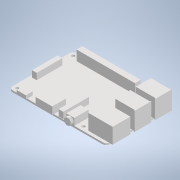
# Autodesk Inventor part: RaspberryPi3B_Mockup
Saved by Autodesk Inventor 2021 (Build 250183000, 183)
## iProperties
Created: 2021-04-19
Part Number: RaspberryPi3B_Mockup
Material: Generic
Document SubType Name: Modeling
Designer: trent
Density: 1 g/cm^3
Appearance: Default
Author: trent
Autodesk Inventor part; units mm, degrees
ref_plane "YZ Plane" through (0, 0, 0) normal (1, 0, 0) x (0, 1, 0)
ref_plane "XZ Plane" through (0, 0, 0) normal (0, 1, 0) x (-1, 0, 0)
ref_plane "XY Plane" through (0, 0, 0) normal (0, 0, 1) x (1, 0, 0)
sketch "Sketch1" plane through (0, 0, 0) normal (0, 1, 0) x (-1, 0, 0)
  line L0 (-3, 0) -> (-82, 0)
  line L1 (-85, -3) -> (-85, -53)
  line L2 (-82, -56) -> (-3, -56)
  line L3 (0, -53) -> (0, -3)
  arc A0 (-3, -56) -> (0, -53) centre (-3, -53) ccw
  arc A1 (0, -3) -> (-3, 0) centre (-3, -3) ccw
  arc A2 (-82, 0) -> (-85, -3) centre (-82, -3) ccw
  arc A3 (-85, -53) -> (-82, -56) centre (-82, -53) ccw
  circle A4 centre (-3.5, -52.5) radius 1.35
  circle A5 centre (-3.5, -3.5) radius 1.35
  circle A6 centre (-61.5, -52.5) radius 1.35
  circle A7 centre (-61.5, -3.5) radius 1.35
  point P0 (0, 0)
  point P1 (-85, -56)
  point P2 (-85, 0)
  point P3 (0, -56)
  dimension "d0" = 85
  dimension "d1" = 56
  dimension "d2" = 3
  dimension "d9" = 2.7
  dimension "d10" = 2.7
  dimension "d15" = 2.7
  dimension "d16" = 2.7
  dimension "d140" = 58
  dimension "d141" = 58
  dimension "d142" = 49
  dimension "d143" = 3.5
  constraints: 8 centre point, 8 end point, 8 point on circle, 8 point on line, 8 tangent, 3 equal radius, 2 parallel, 1 horizontal, 1 perpendicular
  measures "d0" distance of point (-85, -56) point (0, -56)
  measures "d1" distance of point (-85, 0) point (-85, -56)
  measures "d2" radius of A0
  measures "d9" diameter of A4
  measures "d10" diameter of A5
  measures "d15" diameter of A6
  measures "d16" diameter of A7
  measures "d140" distance of A6.centre A4.centre
  measures "d141" distance of A5.centre A7.centre
  measures "d142" distance of A4.centre A5.centre
  measures "d143" distance from line of L0 A5.centre
extrude "Extrusion1" add sketch "Sketch1" along normal blind 1.5
sketch "Sketch2" plane through (0, 1.5, 0) normal (0, 1, 0) x (1, 0, 0)
  circle A0 centre (3.5, 3.5) radius 1.35 projected
  circle A1 centre (3.5, 3.5) radius 3
  circle A2 centre (3.5, 52.5) radius 1.35 projected
  circle A3 centre (3.5, 52.5) radius 3
  circle A4 centre (61.5, 52.5) radius 1.35 projected
  circle A5 centre (61.5, 52.5) radius 3
  circle A6 centre (61.5, 3.5) radius 1.35 projected
  circle A7 centre (61.5, 3.5) radius 3
  point P0 (0, 0)
  dimension "d19" = 6
  dimension "d20" = 6
  dimension "d21" = 6
  dimension "d22" = 6
  constraints: 4 centre point, 4 coincident
  measures "d19" diameter of A1
  measures "d20" diameter of A3
  measures "d21" diameter of A5
  measures "d22" diameter of A7
extrude "Extrusion2" cut sketch "Sketch2" against normal blind 0.001 contours A0 | A1 | A3 | A5 | A6 | A7
sketch "Sketch3" plane through (0, 1.5, 0) normal (0, 1, 0) x (1, 0, 0)
  line L0 (7.25, 55) -> (58.25, 55)
  line L1 (58.25, 55) -> (58.25, 50)
  line L2 (58.25, 50) -> (7.25, 50)
  line L3 (7.25, 50) -> (7.25, 55)
  line L4 (32.75, 55) -> (32.75, 50)
  line L5 (32.75, 52.5) -> (7.25, 52.5)
  line L6 (0, 53) -> (0, 3) projected
  line L7 (82, 56) -> (3, 56) projected
  circle A0 centre (3.5, 52.5) radius 1.35 projected
  point P0 (0, 0)
  dimension "d25" = 51
  dimension "d26" = 5
  dimension "d28" = 25.5
  dimension "d29" = 2.5
  dimension "d30" = 3.5
  dimension "d152" = 7.25
  constraints: 12 end point, 4 midpoint, 2 parallel, 1 horizontal, 1 perpendicular
  measures "d25" distance of L0.start L0.end
  measures "d26" distance of L0.end L1.end
  measures "d28" distance between parallel lines of L4 L3
  measures "d29" distance between parallel lines of L0 L5
  measures "d30" distance between parallel lines of L7 L5
  measures "d152" distance between parallel lines of L6 L3
extrude "Extrusion3" add sketch "Sketch3" along normal blind 8.75 contours L0 L4 L5 L3 | L0 L1 L2 L4 | L5 L4 L2 L3
sketch "Sketch4" plane through (0, 1.5, 0) normal (0, 1, 0) x (1, 0, 0)
  line L0 (1.95, 18.15) -> (6.05, 18.15)
  line L1 (6.05, 18.15) -> (6.05, 40.55)
  line L2 (6.05, 40.55) -> (1.95, 40.55)
  line L3 (1.95, 40.55) -> (1.95, 18.15)
  line L4 (4, 40.55) -> (4, 18.15)
  line L5 (1.95, 29.35) -> (6.05, 29.35)
  line L6 (0, 53) -> (0, 3) projected
  circle A0 centre (3.5, 3.5) radius 1.35 projected
  point P0 (0, 0)
  dimension "d34" = 4.1
  dimension "d35" = 22.4
  dimension "d36" = 4
  dimension "d37" = 24.5
  constraints: 12 end point, 4 midpoint, 2 parallel, 1 horizontal, 1 perpendicular
  measures "d34" distance of L1.end L2.end
  measures "d35" distance of L0.end L1.end
  measures "d36" distance between parallel lines of L6 L4
  measures "d37" distance edge to line of A0 L5
extrude "Extrusion4" add sketch "Sketch4" along normal blind 5.5 contours L3 L5 L4 L0 | L4 L5 L1 L0 | L3 L2 L4 L5 | L4 L2 L1 L5
sketch "Sketch5" plane through (0, 1.5, 0) normal (0, 1, 0) x (1, 0, 0)
  line L0 (7.93, 4.71) -> (15.97, 4.71)
  line L1 (15.97, 4.71) -> (15.97, -1.22)
  line L2 (15.97, -1.22) -> (7.93, -1.22)
  line L3 (7.93, -1.22) -> (7.93, 4.71)
  line L4 (3, 0) -> (82, 0) projected
  line L5 (11.95, -1.22) -> (11.95, 4.71)
  circle A0 centre (3.5, 3.5) radius 1.35 projected
  point P0 (0, 0)
  dimension "d44" = 1.22
  dimension "d45" = 5.93
  dimension "d46" = 8.04
  dimension "d74" = 7.1
  constraints: 10 end point, 2 midpoint, 2 parallel, 1 horizontal, 1 perpendicular
  measures "d44" distance between parallel lines of L2 L4
  measures "d45" distance of L2.end L0.start
  measures "d46" distance of L1.end L2.end
  measures "d74" distance edge to line of A0 L5
extrude "Extrusion5" add sketch "Sketch5" along normal blind 3.2 contours L0 L5 L4 L3 | L0 L1 L4 L5 | L4 L5 L2 L3 | L4 L1 L2 L5
sketch "Sketch6" plane through (0, 1.5, 0) normal (0, 1, 0) x (1, 0, 0)
  line L0 (7.93, -1.22) -> (15.97, -1.22) projected
  line L1 (11.95, -1.22) -> (11.95, 4.71)
  line L2 (7.93, 4.71) -> (15.97, 4.71) projected
  line L3 (24.75, 10.65) -> (39.25, 10.65)
  line L4 (39.25, 10.65) -> (39.25, -1.5)
  line L5 (39.25, -1.5) -> (24.75, -1.5)
  line L6 (24.75, -1.5) -> (24.75, 10.65)
  line L7 (15.97, 0) -> (82, 0) projected
  circle A0 centre (3.5, 3.5) radius 1.35 projected
  line L8 (0, 53) -> (0, 3) projected
  point P0 (0, 0)
  dimension "d144" = 14.5
  dimension "d145" = 12.15
  dimension "d146" = 1.5
  dimension "d153" = 24.75
  constraints: 10 end point, 2 midpoint, 2 parallel, 1 horizontal, 1 perpendicular
  measures "d144" distance of L4.end L5.end
  measures "d145" distance of L3.end L4.end
  measures "d146" distance between parallel lines of L5 L7
  measures "d153" distance between parallel lines of L8 L6
extrude "Extrusion6" add sketch "Sketch6" along normal blind 6.5 contours L3 L4 L7 L6 | L7 L4 L5 L6
sketch "Sketch7" plane through (0, 1.5, 0) normal (0, 1, 0) x (1, 0, 0)
  line L0 (1.95, 40.55) -> (1.95, 18.15) projected
  line L1 (6.05, 18.15) -> (6.05, 40.55) projected
  line L2 (42.95, 22.7) -> (47.05, 22.7)
  line L3 (47.05, 22.7) -> (47.05, 0.3)
  line L4 (47.05, 0.3) -> (42.95, 0.3)
  line L5 (42.95, 0.3) -> (42.95, 22.7)
  line L6 (45, 0.3) -> (45, 22.7)
  line L7 (42.95, 11.5) -> (47.05, 11.5)
  line L8 (0, 53) -> (0, 3) projected
  point P0 (0, 0)
  dimension "d78" = 4.1
  dimension "d80" = 22.4
  dimension "d150" = 45
  constraints: 12 end point, 4 midpoint, 2 parallel, 1 horizontal, 1 perpendicular
  measures "d78" distance of L2.start L2.end
  measures "d80" distance of L0.start L0.end
  measures "d150" distance between parallel lines of L8 L6
extrude "Extrusion7" add sketch "Sketch7" along normal blind 5.5
sketch "Sketch8" plane through (0, 1.5, 0) normal (0, 1, 0) x (1, 0, 0)
  line L0 (50, 0) -> (57, 0)
  line L1 (57, 0) -> (57, 12.5)
  line L2 (57, 12.5) -> (50, 12.5)
  line L3 (50, 12.5) -> (50, 0)
  line L4 (50, 6.25) -> (57, 6.25)
  line L5 (53.5, 0) -> (53.5, 12.5)
  line L6 (3, 0) -> (82, 0) projected
  line L7 (47.05, 0.3) -> (42.95, 0.3) projected
  line L8 (45, 0.3) -> (45, 22.7)
  line L9 (42.95, 22.7) -> (47.05, 22.7) projected
  circle A0 centre (3.5, 3.5) radius 1.35 projected
  line L10 (0, 53) -> (0, 3) projected
  point P0 (0, 0)
  point P1 (43.35, 0)
  dimension "d85" = 7
  dimension "d86" = 12.5
  dimension "d89" = 0
  dimension "d149" = 53.5
  constraints: 14 end point, 6 midpoint, 2 parallel, 1 horizontal, 1 perpendicular
  measures "d85" distance of L1.end L2.end
  measures "d86" distance of L0.end L1.end
  measures "d89" distance between parallel lines of L6 L0
  measures "d149" distance between parallel lines of L10 L5
extrude "Extrusion8" add sketch "Sketch8" along normal blind 6 contours L3 L4 L5 L0 | L5 L4 L1 L0 | L3 L2 L5 L4 | L5 L2 L1 L4
sketch "Sketch9" plane through (3, 0, 0) normal (0, 0, 1) x (1, 0, 0)
  line L0 (54, 7.5) -> (47, 7.5) projected
  line L1 (54, 1.5) -> (54, 7.5) projected
  circle A0 centre (50.5, 4.25) radius 3
  point P0 (-3, 0)
  dimension "d96" = 3.5
  dimension "d97" = 3.25
  dimension "d98" = 6
  constraints: 1 centre point
  measures "d96" distance from line of L1 A0.centre
  measures "d97" distance from line of L0 A0.centre
  measures "d98" diameter of A0
extrude "Extrusion9" add sketch "Sketch9" along normal blind 2.5
sketch "Sketch10" plane through (0, 1.5, 0) normal (0, 1, 0) x (1, 0, 0)
  line L0 (66.65, 18) -> (88, 18)
  line L1 (88, 18) -> (88, 2.5)
  line L2 (88, 2.5) -> (66.65, 2.5)
  line L3 (66.65, 2.5) -> (66.65, 18)
  line L4 (85, 3) -> (85, 53) projected
  line L5 (88, 10.25) -> (66.65, 10.25)
  line L6 (57, 0) -> (82, 0) projected
  point P0 (0, 0)
  dimension "d101" = 21.35
  dimension "d102" = 15.5
  dimension "d103" = 3
  dimension "d104" = 10.25
  constraints: 10 end point, 2 midpoint, 2 parallel, 1 horizontal, 1 perpendicular
  measures "d101" distance of L0.start L0.end
  measures "d102" distance of L2.end L0.start
  measures "d103" distance between parallel lines of L1 L4
  measures "d104" distance between parallel lines of L6 L5
extrude "Extrusion10" add sketch "Sketch10" along normal blind 13.5
sketch "Sketch11" plane through (0, 1.5, 0) normal (0, 1, 0) x (1, 0, 0)
  line L0 (70.3341, 22.43) -> (87.5, 22.43)
  line L1 (88, 2.4833) -> (88, 15.6315)
  line L2 (87.5, 35.57) -> (70.3341, 35.57)
  line L3 (70.3341, 35.57) -> (70.3341, 22.43)
  line L4 (85, 3) -> (85, 53) projected
  line L5 (88, 36.35) -> (87.5, 36.35)
  line L6 (87.5, 21.65) -> (88, 21.65)
  line L7 (88, 21.65) -> (88, 36.35)
  line L8 (87.5, 36.35) -> (87.5, 35.57)
  line L9 (87.5, 22.43) -> (87.5, 21.65)
  line L10 (88, 29) -> (70.3341, 29)
  line L11 (70.3, 40.43) -> (87.5, 40.43)
  line L12 (88, 22.6143) -> (88, 34.7304)
  line L13 (87.5, 53.57) -> (70.3, 53.57)
  line L14 (70.3, 53.57) -> (70.3, 40.43)
  line L15 (88, 54.35) -> (87.5, 54.35)
  line L16 (87.5, 39.65) -> (88, 39.65)
  line L17 (88, 39.65) -> (88, 54.35)
  line L18 (87.5, 54.35) -> (87.5, 53.57)
  line L19 (87.5, 40.43) -> (87.5, 39.65)
  line L20 (88, 47) -> (70.3, 47)
  line L21 (66.65, 2.5) -> (66.65, 18) projected
  line L22 (66.65, 10.25) -> (88, 10.25)
  line L23 (57, 0) -> (82, 0) projected
  point P0 (0, 0)
  point P1 (85, 38)
  point P2 (88, 34.35)
  dimension "d107" = 3
  dimension "d109" = 13.14
  dimension "d113" = 14.7
  dimension "d115" = 13.14
  dimension "d119" = 14.7
  dimension "d123" = 29
  dimension "d125" = 14.7
  dimension "d126" = 3
  dimension "d127" = 3
  dimension "d129" = 2.5
  dimension "d130" = 2.5
  dimension "d131" = 2.5
  dimension "d132" = 14.6659
  dimension "d133" = 3
  dimension "d134" = 34.7304
  dimension "d135" = 22.6143
  dimension "d136" = 15.6315
  dimension "d137" = 2.4833
  dimension "d151" = 47
  constraints: 42 end point, 10 parallel, 6 perpendicular, 5 horizontal, 5 midpoint
  measures "d107" distance between parallel lines of L1 L4
  measures "d109" distance of L2.end L0.start
  measures "d113" distance of L6.end L5.start
  measures "d115" distance of L14.start L14.end
  measures "d119" distance of L16.end L15.start
  measures "d123" distance between parallel lines of L23 L10
  measures "d125" distance between parallel lines of L4 L14
  measures "d126" distance between parallel lines of L17 L4
  measures "d127" distance between parallel lines of L7 L4
  measures "d129" distance between parallel lines of L19 L4
  measures "d130" distance between parallel lines of L8 L4
  measures "d131" distance between parallel lines of L9 L4
  measures "d132" distance between parallel lines of L3 L4
  measures "d133" distance from line of L22.end L4
  measures "d134" distance from line of L12.end L23
  measures "d135" distance from line of L12.start L23
  measures "d136" distance from line of L1.end L23
  measures "d137" distance from line of L1.start L23
  measures "d151" distance between parallel lines of L23 L20
extrude "Extrusion11" add sketch "Sketch11" along normal blind 16
body "Solid1"
